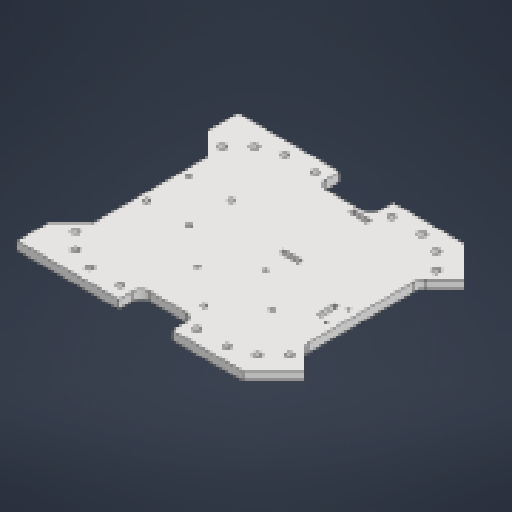
# Autodesk Inventor part: electronics panel
Saved by Autodesk Inventor 2023 (Build 270158000, 158)
## iProperties
Created: 2023-01-16
Part Number: electronics panel
Material: Generic
Document SubType Name: Modeling
Designer: Michael
Density: 1 g/cm^3
Appearance: Default
Author: Michael
Autodesk Inventor part; units mm, degrees
ref_plane "YZ Plane" through (0, 0, 0) normal (1, 0, 0) x (0, 1, 0)
ref_plane "XZ Plane" through (0, 0, 0) normal (0, 1, 0) x (-1, 0, 0)
ref_plane "XY Plane" through (0, 0, 0) normal (0, 0, 1) x (1, 0, 0)
sketch "Sketch2" plane through (0, 0, 0) normal (0, 1, 0) x (-1, 0, 0)
  line L0 (0, 0) -> (152.4, 0)
  line L1 (152.4, 0) -> (152.4, -127)
  line L2 (152.4, -127) -> (0, -127)
  line L3 (0, -127) -> (0, 0)
  line L4 (152.4, -63.5) -> (0, -63.5)
  line L5 (76.2, -127) -> (76.2, 0)
  line L6 (152.4, -104.4927) -> (130.0062, -127)
  line L7 (130.0062, -127) -> (146.1909, -143.1442)
  line L8 (146.1909, -143.1442) -> (168.6133, -120.6655)
  line L9 (168.6133, -120.6655) -> (152.4, -104.4927)
  line L10 (0, -104.4927) -> (22.3938, -127)
  line L11 (22.3938, -127) -> (6.2091, -143.1442)
  line L12 (6.2091, -143.1442) -> (-16.2133, -120.6655)
  line L13 (-16.2133, -120.6655) -> (0, -104.4927)
  line L14 (152.4, -22.5073) -> (130.0062, 0)
  line L15 (130.0062, 0) -> (146.1909, 16.1442)
  line L16 (146.1909, 16.1442) -> (168.6133, -6.3345)
  line L17 (168.6133, -6.3345) -> (152.4, -22.5073)
  line L18 (6.2091, 16.1442) -> (-16.2133, -6.3345)
  line L19 (-16.2133, -6.3345) -> (0, -22.5073)
  line L20 (0, -22.5073) -> (22.3938, 0)
  line L21 (22.3938, 0) -> (6.2091, 16.1442)
  line L22 (168.6133, -120.6655) -> (168.6133, -143.1442)
  line L23 (168.6133, -143.1442) -> (146.1909, -143.1442)
  line L24 (-16.2133, -120.6655) -> (-16.2133, -143.1442)
  line L25 (-16.2133, -143.1442) -> (6.2091, -143.1442)
  line L26 (168.6133, -6.3345) -> (168.6133, 16.1442)
  line L27 (168.6133, 16.1442) -> (146.1909, 16.1442)
  line L28 (-16.2133, 16.1442) -> (6.2091, 16.1442)
  line L29 (-16.2133, -6.3345) -> (-16.2133, 16.1442)
  line L30 (146.1909, -143.1442) -> (95.3909, -143.1442)
  line L31 (95.3909, -143.1442) -> (95.3909, -127)
  line L32 (0, -63.5) -> (152.4, -63.5)
  line L33 (6.2091, -143.1442) -> (57.0091, -143.1442)
  line L34 (57.0091, -143.1442) -> (57.0091, -127)
  line L35 (146.1909, 16.1442) -> (95.3909, 16.1442)
  line L36 (95.3909, 16.1442) -> (95.3909, 0)
  line L37 (6.2091, 16.1442) -> (57.0091, 16.1442)
  line L38 (57.0091, 16.1442) -> (57.0091, 0)
  point P0 (0, -22.4519)
  point P1 (22.4494, 0)
  point P2 (22.4494, -127)
  point P3 (0, -104.5481)
  point P4 (95.3909, 0)
  point P5 (152.4, -22.5073)
  point P6 (0, -22.5073)
  point P7 (57.0091, 0)
  point P8 (0, -104.4927)
  point P9 (160.5067, -112.5791)
  point P10 (160.5067, -14.4209)
  point P11 (130.0062, 0)
  point P12 (130.0062, 0)
  dimension "d0" = 152.4
  dimension "d1" = 127
  dimension "d167" = 31.75
  dimension "d169" = 22.86
  dimension "d170" = 50.8
  constraints: 78 end point, 23 symmetric about line, 6 midpoint, 5 perpendicular, 3 point on line, 2 horizontal, 2 parallel, 1 vertical
  measures "d0" distance of L1.end L2.end
  measures "d1" distance of L0.end L1.end
  measures "d167" distance of L6.start L6.end
  measures "d169" distance of L6.end L7.end
  measures "d170" distance of L7.end L30.end
extrude "Extrusion8" add sketch "Sketch2" against normal blind 6.35 contours L3 L19 L18 L21 L0 | L0 L20 L3 | L21 L37 L38 L0 | L0 L5 L4 L3 L20 | L4 L5 L2 L10 L3 | L0 L14 L1 L4 L5 | L10 L2 L3 | L3 L2 L11 L12 L13 | L4 L1 L6 L2 L5 | L36 L35 L15 L0 | L2 L34 L33 L11 | L15 L16 L17 L1 L0 | L0 L1 L14 | L9 L8 L7 L2 L1 | L1 L2 L6 | L2 L7 L30 L31 | L27 L26 L16 | L22 L23 L8
sketch "Sketch14" plane through (0, 0, 0) normal (0, 1, 0) x (1, 0, 0)
  line L0 (0, 0) -> (0, 104.4927) projected
  line L1 (0, 104.4927) -> (0, 0) projected
  line L2 (0, 52.2463) -> (-12.6589, 52.2463)
  line L3 (0, 23.7671) -> (-12.6589, 23.7671)
  arc A0 (0.9301, 105.4781) -> (0, 103.2329) centre (3.175, 103.2329) ccw projected
  line L4 (0, 103.2329) -> (-12.6589, 103.2329)
  point P0 (-6.3246, 44.3088)
  point P1 (-6.3295, 52.2463)
  point P2 (-6.3246, 60.1838)
  point P3 (0, 127)
  dimension "d89" = 7.9375
  dimension "d90" = 6.3246
  constraints: 6 end point, 3 horizontal, 2 midpoint, 1 symmetric about line
  measures "d89" distance of point (-6.329, 52.246) point (-6.325, 44.309)
  measures "d90" distance from line of L0 point (-6.325, 44.309)
hole "Hole3" at (-6.3246, 0, -44.3088) at (-6.3246, 0, -60.1838) direction (0, -1, 0) diameter 1.5999 end through all
sketch "Sketch16" plane through (0, 0, 0) normal (0, 1, 0) x (1, 0, 0)
  point P0 (0, 0)
  point P1 (-146.6643, 55.3769)
  point P2 (-147.0122, 85.8749)
  point P3 (-116.5122, 85.9271)
  point P4 (-116.1643, 55.4291)
  dimension "d109" = 30.5
  dimension "d110" = 30.5
  dimension "d111" = 30.5
  dimension "d112" = 30.5
  dimension "d172" = 43.3421
  dimension "d173" = 42.924
  measures "d109" distance of point (-147.012, 85.875) point (-146.664, 55.377)
  measures "d110" distance of point (-116.512, 85.927) point (-116.164, 55.429)
  measures "d111" distance of point (-116.164, 55.429) point (-146.664, 55.377)
  measures "d112" distance of point (-116.512, 85.927) point (-147.012, 85.875)
  measures "d172" distance of point (-116.164, 55.429) point (-147.012, 85.875)
  measures "d173" distance of point (-116.512, 85.927) point (-146.664, 55.377)
hole "Hole5" at (-146.6643, 0, -55.3769) at (-147.0122, 0, -85.8749) at (-116.5122, 0, -85.9271) at (-116.1643, 0, -55.4291) direction (0, -1, 0) diameter 4 end through all
sketch "Sketch17" plane through (0, 0, 0) normal (0, 1, 0) x (1, 0, 0)
  line L0 (-127.2393, 115.3557) -> (-127.2393, 74.7157) projected
  line L1 (-127.2393, 74.7157) -> (-51.0393, 74.7157) projected
  line L2 (-51.0393, 74.7157) -> (-51.0393, 115.3557) projected
  line L3 (-51.0393, 115.3557) -> (-127.2393, 115.3557) projected
  line L4 (-57.0091, 127) -> (-95.3909, 127) projected
  line L5 (-95.3909, 127) -> (-57.0091, 127) projected
  line L6 (-60.2753, 120.839) -> (-66.6253, 120.839)
  line L7 (-66.6253, 120.839) -> (-66.6253, 124.014)
  line L8 (-66.6253, 124.014) -> (-60.2753, 124.014)
  line L9 (-60.2753, 124.014) -> (-60.2753, 120.839)
  line L10 (-60.2753, 120.839) -> (-53.9253, 120.839)
  line L11 (-53.9253, 120.839) -> (-53.9253, 124.014)
  line L12 (-53.9253, 124.014) -> (-60.2753, 124.014)
  line L13 (-60.2753, 124.014) -> (-60.2753, 120.839)
  line L14 (-60.2753, 71.0389) -> (-66.6253, 71.0389)
  line L15 (-66.6253, 71.0389) -> (-66.6253, 74.2139)
  line L16 (-66.6253, 74.2139) -> (-60.2753, 74.2139)
  line L17 (-60.2753, 74.2139) -> (-60.2753, 71.0389)
  line L18 (-60.2753, 71.0389) -> (-53.9253, 71.0389)
  line L19 (-53.9253, 71.0389) -> (-53.9253, 74.2139)
  line L20 (-53.9253, 74.2139) -> (-60.2753, 74.2139)
  line L21 (-60.2753, 74.2139) -> (-60.2753, 71.0389)
  line L22 (-57.0091, 143.1442) -> (-57.0091, 127) projected
  point P0 (0, 0)
  point P1 (-70.5279, 127)
  point P2 (-107.2721, 127)
  point P3 (-87.3125, 128.5875)
  point P4 (0, 127)
  point P5 (-127, 127)
  dimension "d120" = 6.35
  dimension "d121" = 3.175
  dimension "d122" = 6.35
  dimension "d123" = 6.35
  dimension "d124" = 3.175
  dimension "d125" = 6.35
  constraints: 32 end point, 8 parallel, 4 horizontal, 4 perpendicular, 2 point on line
  measures "d120" distance of L7.end L8.end
  measures "d121" distance of L6.end L7.end
  measures "d122" distance of L12.end L11.end
  measures "d123" distance of L15.end L17.start
  measures "d124" distance of L14.end L15.end
  measures "d125" distance of L20.end L20.start
extrude "Extrusion14" cut sketch "Sketch17" against normal blind 11.1125 contours L6 L7 L8 L9 | L9 L12 L11 L10 | L14 L15 L16 L17 | L17 L20 L19 L18
sketch "Sketch18" plane through (0, 0, 0) normal (0, 1, 0) x (1, 0, 0)
  circle A0 centre (-60.5524, 54.6756) radius 1.6
  circle A1 centre (-87.5891, 32.6757) radius 1.6
  circle A2 centre (-33.5891, 32.6757) radius 1.6
  circle A3 centre (-60.5524, 10.6757) radius 1.6076
  point P0 (0, 0)
  constraints: 4 centre point, 8 other
sketch "Sketch19" plane through (0, 0, 0) normal (0, 1, 0) x (1, 0, 0)
  line L0 (-14.8408, 45.8963) -> (-11.6658, 45.8963)
  line L1 (-11.6658, 45.8963) -> (-11.6658, 58.5963)
  line L2 (-11.6658, 58.5963) -> (-14.8408, 58.5963)
  line L3 (-14.8408, 58.5963) -> (-14.8408, 45.8963)
  circle A0 centre (-6.3246, 44.3088) radius 0.8 projected
  circle A1 centre (-6.3246, 60.1838) radius 0.8 projected
  line L4 (-6.3246, 44.3088) -> (-14.8408, 44.3088)
  circle A2 centre (-6.3246, 60.1838) radius 0.8 projected
  line L5 (-6.3246, 60.1838) -> (-14.8408, 60.1838)
  point P0 (0, 0)
  point P1 (-13.2533, 45.8963)
  dimension "d130" = 3.175
  dimension "d131" = 12.7
  dimension "d132" = 1.5875
  constraints: 12 end point, 3 horizontal, 2 parallel, 1 midpoint, 1 perpendicular
  measures "d130" distance of L2.end L1.end
  measures "d131" distance of L1.end L0.end
  measures "d132" distance from line of L4 point (-13.253, 45.896)
extrude "Extrusion16" cut sketch "Sketch19" against normal blind 25.4 contours L3 L2 L1 L0
sketch "Sketch23" plane through (0, 0, 0) normal (0, 1, 0) x (1, 0, 0)
  line L0 (-95.3909, 127) -> (-57.0091, 127) projected
  line L1 (-76.2, 127) -> (-76.2, 96.1497)
  line L2 (-152.4, 22.5073) -> (-152.4, 104.4927) projected
  line L3 (-152.4, 63.5) -> (-115.4965, 63.5)
  line L4 (-95.3909, 143.1442) -> (-168.6133, 143.1442) projected
  line L5 (-95.3909, 127) -> (-95.3909, 143.1442) projected
  point P0 (-177.8, 23.7671)
  point P1 (-177.8, 103.2329)
  point P2 (-103.7729, 133.6192)
  point P3 (-125.6156, 133.6192)
  point P4 (-48.6271, 133.6192)
  point P5 (-26.7844, 133.6192)
  point P6 (-103.7729, -6.6192)
  point P7 (-103.7729, -6.6192)
  point P8 (-125.6156, -6.6192)
  point P9 (-48.6271, -6.6192)
  point P10 (-26.7844, -6.6192)
  point P11 (-132.0021, 143.1442)
  dimension "d185" = 21.8427
  dimension "d186" = 9.525
  dimension "d187" = 9.525
  dimension "d190" = 8.382
  constraints: 6 symmetric about line, 4 end point, 3 midpoint, 1 coincident, 1 horizontal, 1 vertical
  measures "d185" distance of point (-103.773, 133.619) point (-125.616, 133.619)
  measures "d186" distance from line of L4 point (-103.773, 133.619)
  measures "d187" vertical distance of point (-132.002, 143.144) point (-125.616, 133.619)
  measures "d190" distance from line of L5 point (-103.773, 133.619)
extrude "Extrusion18" cut sketch "Sketch18" against normal blind 6.35
sketch "Sketch24" plane through (0, 0, 0) normal (0, 1, 0) x (1, 0, 0)
  circle A0 centre (0.8987, 116.2224) radius 2.4765
  circle A1 centre (-10.775, 127.8974) radius 2.4765
  circle A2 centre (0.8987, 10.7776) radius 2.4765
  circle A3 centre (-10.775, -0.8974) radius 2.4765
  circle A4 centre (-141.625, 127.8974) radius 2.4765
  circle A5 centre (-153.2987, 116.2224) radius 2.4765
  circle A6 centre (-153.2987, 10.7776) radius 2.4765
  circle A7 centre (-141.625, -0.8974) radius 2.4765
  point P0 (0, 0)
  constraints: 8 centre point, 16 other
extrude "Extrusion19" cut sketch "Sketch24" against normal blind 6.35
hole "Hole9" at (-103.7729, 0, -133.6192) at (-125.6156, 0, -133.6192) at (-48.6271, 0, -133.6192) at (-26.7844, 0, -133.6192) at (-48.6271, 0, 6.6192) at (-26.7844, 0, 6.6192) at (-125.6156, 0, 6.6192) at (-103.7729, 0, 6.6192) direction (0, -1, 0) diameter 4.953 depth 10.414
fillet "Fillet5" radius 6.35 6 edges at (-57.0091, -3.175, -127) (-95.3909, -3.175, -127) (-57.0091, -3.175, 0) (-95.3909, -3.175, 0) (0, -3.175, -22.5073) (0, -3.175, -104.4927)
sketch "Sketch25" plane through (16.2133, -6.35, -120.6655) normal (0.7079924, 0, -0.7062201) x (-0.7062201, 0, -0.7079924)
  ellipse E0 centre (7.1969, 3.175) end of major axis (7.1969, 1.975) minor radius 1.2
  ellipse E1 centre (24.5108, 3.175) end of major axis (24.5108, 1.975) minor radius 1.2
  point P0 (-73.98, 6.35)
  constraints: 2 centre point, 2 coincident, 4 other
hole "Hole10" at (11.1307, -3.175, -125.7608) at (-1.0967, -3.175, -138.0189) direction (-0.7079924, 0, 0.7062201) diameter 1.6 depth 10.414
sketch "Sketch26" plane through (-6.2091, -6.35, 16.1442) normal (0.7079924, 0, 0.7062201) x (0.7062201, 0, -0.7079924)
  ellipse E0 centre (7.124, 3.175) end of major axis (7.124, 1.975) minor radius 1.2
  ellipse E1 centre (24.4378, 3.175) end of major axis (24.4378, 1.975) minor radius 1.2
  point P0 (15.815, 6.35)
  constraints: 2 centre point, 2 coincident, 4 other
hole "Hole11" at (-1.178, -3.175, 11.1005) at (11.0494, -3.175, -1.1576) direction (-0.7079924, 0, -0.7062201) diameter 1.6 depth 10.414
body "Solid3"
